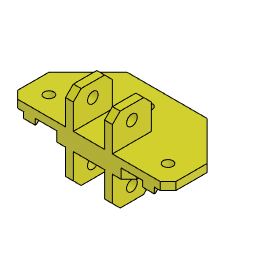
Bed Lift Idler Buddy_2x (Autodesk Fusion 360 design; units mm, degrees)
Autodesk Fusion 360 part; units mm, degrees
note: some values were not read from the file. Set by a fixed rule: the direction of a hole.
sketch "Sketch1" plane through (207.95, 134, 0) normal (0, 0, 1) x (1, 0, 0)
  line L0 (-207.95, -120) -> (-126.95, -120)
  line L1 (-126.95, -120) -> (-126.95, -134)
  line L2 (-126.95, -134) -> (-207.95, -134)
  line L3 (-207.95, -134) -> (-207.95, -120)
  line L4 (-167.45, -134) -> (-167.45, -146) construction
  line L5 (-167.45, -140) -> (-164.45, -140) construction
  line L6 (-167.45, -140) -> (-55.6884, -140)
  line L7 (-55.6884, -137.5) -> (-55.6884, -142.5)
  line L8 (-146.95, -120) -> (-146.95, -134)
  line L9 (-187.95, -120) -> (-187.95, -134)
  point P0 (-167.45, -134)
  point P1 (-207.95, -134)
  constraint horizontal L0
  constraint vertical L1
  constraint horizontal L2
  constraint vertical L3
  constraint midpoint L2 P0
  constraint vertical L4
  constraint coincident P0 L4.start
  constraint horizontal L5
  constraint midpoint L4 L5.start
  constraint perpendicular L4 L6
  constraint vertical L7
  constraint midpoint L6.end L7
  constraint coincident L0 L8.start
  constraint coincident L2 L8.end
  constraint perpendicular L2 L8
  constraint coincident L0 L9.start
  constraint coincident L2 L9.end
  constraint perpendicular L2 L9
  constraint coincident P1 L2.end
  measures "d6013" distance of L0.start L0.end
  measures "d6014" distance of L0.start L2.end
  measures "d6017" distance of P0 L4.end
  measures "d6018" distance of L5.start L5.end
  measures "d6019" distance of L7.start L7.end
  measures "d6020" distance of P1 L9.end
  measures "d6021" distance of L1.end L8.end
extrude "Extrude1" add sketch "Sketch1" along normal blind 4
extrude "Extrude2" add sketch "Sketch1" against normal blind 5 contours L0 L2 L8 L9
sketch "Sketch4" plane through (0, 14, 0) normal (0, 1, 0) x (-1, 0, 0)
  line L0 (-61, -5) -> (-20, -5)
  line L1 (-20, -5) -> (-20, 0)
  line L2 (-20, 0) -> (0, 0)
  line L3 (0, 4) -> (-81, 4)
  line L4 (-81, 0) -> (-61, 0)
  line L5 (-61, 0) -> (-61, -5)
  line L6 (0, 0) -> (0, 4)
  line L7 (-81, 4) -> (-81, 0)
  line L8 (-40.5, 4) -> (-40.5, -5) construction
  line L9 (-28.5, -22) -> (-52.5, -22)
  line L10 (-52.5, -22) -> (-52.5, -5)
  line L11 (-52.5, -5) -> (-28.5, -5)
  line L12 (-28.5, -5) -> (-28.5, -22)
  line L13 (-36.25, 234.1382) -> (-44.75, 234.1382) construction
  line L14 (-44.75, 234.1382) -> (-44.75, 246.1382) construction
  line L15 (-44.75, 246.1382) -> (-36.25, 246.1382) construction
  line L16 (-36.25, 246.1382) -> (-36.25, 234.1382) construction
  line L17 (-32.5, -22) -> (-32.5, -5)
  line L18 (-48.5, -5) -> (-48.5, -22)
  line L19 (-61, -0.5) -> (-20, -0.5) construction
  line L20 (-28.5, 4) -> (-28.5, 21)
  line L21 (-28.5, 21) -> (-52.5, 21)
  line L22 (-32.5, 21) -> (-32.5, 4)
  line L23 (-48.5, 4) -> (-48.5, 21)
  line L24 (-52.5, 21) -> (-52.5, 4)
  point P0 (-40.5, -0.5)
  point P1 (-40.5, -0.5)
  dimension "d6225" = 20
  dimension "d6226" = 17
  dimension "d6227" = 8.5
  dimension "d6228" = 12
  dimension "d6229" = 4
  dimension "d6280" = 22
  dimension "d576" = 16
  constraint midpoint L0 L8.end
  constraint midpoint L3 L8.start
  constraint horizontal L9
  constraint vertical L10
  constraint horizontal L11
  constraint vertical L12
  constraint symmetric L8 L9.start L9.end
  constraint horizontal L13
  constraint vertical L14
  constraint horizontal L15
  constraint vertical L16
  constraint symmetric L8 L13.start L13.end
  constraint coincident L9 L17.start
  constraint coincident L11 L17.end
  constraint perpendicular L11 L17
  constraint coincident L11 L18.start
  constraint coincident L9 L18.end
  constraint perpendicular L9 L18
  constraint symmetric L8 L17.start L18.end
  constraint coincident L0 L10.end
  constraint coincident L5 L19.start
  constraint coincident L1 L19.end
  constraint perpendicular L1 L19
  constraint midpoint L19 P1
  constraint midpoint L8 P1
  constraint coincident P1 P0
  constraint symmetric L9.start L19 L20.end
  constraint symmetric L9.end L19 L21.end
  constraint symmetric L10.end L19 L24.end
  constraint symmetric L11.end L19 L20.start
  constraint symmetric L17.start L19 L22.start
  constraint symmetric L17.end L19 L22.end
  constraint symmetric L18.start L19 L23.start
  constraint symmetric L18.end L19 L23.end
  measures "d6226" distance of L9.start L11.end
  measures "d6227" distance of L13.start L13.end
  measures "d6228" distance of L13.start L15.end
  measures "d6229" distance of L10.end L18.start
  measures "d6280" vertical distance of L4.end L9.end
  measures "d576" distance of L17.start L18.end
extrude "Extrude5" add sketch "Sketch4" along normal blind 3 and the other way blind 14 contours L0 L9 L10 L11 L18 | L0 L9 L11 L12 L17 | L3 L21 L23 L24 | L3 L20 L21 L22
hole "Hole5" at (28.5, 10, -15) direction (1, 0, 0) diameter 5.5 depth 55 tip angle 118
hole "Hole6" at (28.5, 10, 14) direction (1, 0, 0) diameter 5.5 depth 25 tip angle 118
sketch "Sketch5" plane through (28.5, 0, 0) normal (-1, 0, 0) x (0, -1, 0)
  circle A0 centre (-10, -15) radius 2.75
  line L0 (0, -5) -> (-14, -5)
  line L1 (-14, -5) -> (-17, -5)
  line L2 (-17, -5) -> (-17, -22)
  line L3 (-17, -22) -> (0, -22)
  line L4 (0, -22) -> (0, -5)
  circle A1 centre (-10, -15) radius 2.75
  circle A2 centre (-10, -15) radius 9 construction
  circle A3 centre (-10, -15) radius 6
  line L5 (-16, -15) -> (-16, 273.6321)
  line L6 (-16, 273.6321) -> (-14, 273.6321)
  line L7 (-14, 0) -> (-14, -5)
  line L8 (-10, -15) -> (-10, -22) construction
  dimension "d6290" = 18
  dimension "d6291" = 12
  dimension "d6292" = 2
  constraint concentric A0 A2
  constraint concentric A1 A3
  constraint coincident A3 L5.start
  constraint tangent A3 L5
  constraint perpendicular L1 L5
  constraint perpendicular L5 L6
  constraint coincident L6.end L7
  constraint coincident A0.centre A1.centre
  constraint coincident L3 L8.end
  constraint perpendicular L3 L8
  measures "d6290" diameter of A2
  measures "d6291" diameter of A3
  measures "d6292" distance of L5.end L6.end
sketch "Sketch6" plane through (0, 14, 0) normal (0, 1, 0) x (-1, 0, 0)
  line L0 (-20, 0) -> (0, 0)
  line L1 (0, 0) -> (0, 4)
  line L2 (0, 4) -> (-28.5, 4)
  line L3 (-28.5, 4) -> (-32.5, 4)
  line L4 (-52.5, 4) -> (-81, 4)
  line L5 (-81, 4) -> (-81, 0)
  line L6 (-81, 0) -> (-61, 0)
  line L7 (-61, 0) -> (-61, -5)
  line L8 (-61, -5) -> (-52.5, -5)
  line L9 (-52.5, -5) -> (-48.5, -5)
  line L10 (-48.5, -5) -> (-32.5, -5)
  line L11 (-32.5, -5) -> (-28.5, -5)
  line L12 (-28.5, -5) -> (-20, -5)
  line L13 (-20, -5) -> (-20, 0)
  line L14 (-61, 0) -> (-61, 4)
  line L15 (-20, 0) -> (-20, 4)
  line L16 (-32.5, 4) -> (-48.5, 4)
  line L17 (-48.5, 4) -> (-52.5, 4)
  constraint coincident L6.end L7.start
  constraint perpendicular L4 L14
  constraint coincident L0.start L13.end
  constraint perpendicular L2 L15
  constraint coincident L4 L14.end
  constraint coincident L2 L15.end
extrude "Extrude6" add sketch "Sketch6" along normal blind 6 contours L0 L1 L2 L15 | L4 L5 L6 L14
hole "Hole7" at (10, 10, 4) direction (0, 0, -1) diameter 5 depth 12 tip angle 180
hole "Hole8" at (71, 10, 4) direction (0, 0, -1) diameter 5 depth 10 tip angle 180
sketch "Sketch8" plane through (0, 20, 0) normal (0, 1, 0) x (-1, 0, 0)
  line L0 (0, 0) -> (0, 4)
  line L1 (0, 4) -> (-20, 4)
  line L2 (-20, 0) -> (0, 0)
  line L3 (-48.5, -5) -> (-48.5, -22)
  line L4 (-48.5, -22) -> (-52.5, -22)
  line L5 (-52.5, -22) -> (-52.5, -5)
  line L6 (-48.5, -5) -> (-32.5, -5)
  line L7 (-32.5, -22) -> (-32.5, -5)
  line L8 (-28.5, -5) -> (-28.5, -22)
  line L9 (-28.5, -22) -> (-32.5, -22)
  line L10 (-28.5, -5) -> (-20, -5)
  line L11 (-20, 0) -> (-20, -5)
  line L12 (-61, 0) -> (-61, -5)
  line L13 (-61, -5) -> (-52.5, -5)
  line L14 (-20, 0) -> (0, 0)
  line L15 (-81, 0) -> (-61, 0)
  line L16 (0, 0) -> (0, 4)
  line L17 (-81, 0) -> (-81, 4)
  line L18 (-10, 0) -> (-10, 4)
  line L19 (-71, 0) -> (-71, 5)
  line L20 (-74, 5) -> (-74, 10)
  line L21 (-74, 10) -> (-68, 10)
  line L22 (-68, 10) -> (-68, 5)
  line L23 (-13.0512, 4) -> (-13.0695, 9)
  line L24 (-7.0712, 9.1427) -> (-6.9488, 4)
  line L25 (-13.0695, 9) -> (-7.0712, 9.1427)
  line L26 (-20, -5) -> (-20, 4)
  line L27 (-24.25, -5) -> (-24.8161, 5.0059)
  line L28 (-61, -5) -> (-61, 5)
  line L29 (-56.75, -5) -> (-56.2231, 5.0071)
  line L30 (-20, 4) -> (-20, 0)
  line L31 (-32.5, 4) -> (-32.5, 21)
  line L32 (-32.5, 21) -> (-28.5, 21)
  line L33 (-28.5, 21) -> (-28.5, 4)
  line L34 (0, 4) -> (-28.5, 4)
  line L35 (-52.5, 4) -> (-52.5, 21)
  line L36 (-52.5, 21) -> (-48.5, 21)
  line L37 (-48.5, 21) -> (-48.5, 4)
  line L38 (-32.5, 4) -> (-48.5, 4)
  line L39 (-52.5, 4) -> (-81, 4)
  dimension "d6767" = 5
  dimension "d6768" = 5
  dimension "d6769" = 6
  dimension "d6770" = 6
  constraint midpoint L14 L18.start
  constraint midpoint L1 L18.end
  constraint midpoint L15 L19.start
  constraint perpendicular L20 L21
  constraint symmetric L19 L20.start L22.end
  constraint coincident L1 L24.end
  constraint symmetric L18 L23.start L24.end
  constraint perpendicular L24 L25
  constraint coincident L10.end L11.end
  constraint coincident L1.end L26.end
  constraint midpoint L10 L27.start
  constraint coincident L12.end L13.start
  constraint midpoint L13 L29.start
  measures "d6767" distance of L20.start L20.end
  measures "d6768" distance of L23.start L23.end
  measures "d6769" distance of L20.end L21.end
  measures "d6770" distance of L23.end L24.start
extrude "Extrude8" add sketch "Sketch8" against normal blind 6 contours L10 L11 L26 L27 L30 L34 | L12 L13 L28 L29 L39
sketch "Sketch9" plane through (0, 0, 0) normal (0, 0, -1) x (1, 0, 0)
  circle A0 centre (71, -10) radius 2.5
  line L0 (61, 0) -> (61, -20)
  line L1 (61, -20) -> (81, -20)
  line L2 (81, -20) -> (81, 0)
  line L3 (81, 0) -> (61, 0)
  circle A1 centre (10, -10) radius 2.5
  line L4 (20, -20) -> (20, 0)
  line L5 (20, 0) -> (0, 0)
  line L6 (0, 0) -> (0, -20)
  line L7 (0, -20) -> (20, -20)
  line L8 (81, -20) -> (81, -40)
  line L9 (81, -40) -> (61, -40)
  line L10 (61, -40) -> (61, -20)
  line L11 (0, -20) -> (0, -40)
  line L12 (0, -40) -> (20, -40)
  line L13 (20, -40) -> (20, -20)
  line L14 (20, -40) -> (81, -40)
  line L15 (81, -40) -> (81, 0)
  line L16 (81, 0) -> (20, 0)
  line L17 (20, 0) -> (20, -40)
  dimension "d305" = 20
  constraint coincident L1.end L2.start
  constraint perpendicular L1 L8
  constraint perpendicular L2 L9
  constraint coincident L0.end L1.start
  constraint perpendicular L1 L10
  constraint coincident L6.end L7.start
  constraint perpendicular L7 L11
  constraint perpendicular L4 L12
  constraint coincident L4.start L7.end
  constraint perpendicular L12 L13
  constraint equal L10 L13
  constraint horizontal L14
  constraint vertical L15
  constraint horizontal L16
  constraint vertical L17
  constraint coincident L2.end L3.start
  measures "d305" distance of L12.end L4.start
extrude "Extrude9" add sketch "Sketch9" against normal blind 4 contours L0 L4 L10 L13 L14 L16 L17 | L1 L8 L9 L10 L14 L15 | L7 L11 L12 L13 L17
hole "Hole9" at (40.469, 30, 0) direction (0, 0, 1) diameter 5 depth 16 tip angle 118
extrude "Extrude10" add 1 faces at (43.1732, 14, -1.6667) along direction (0, 1, 0) blind 6
extrude "Extrude11" add 4 faces at (51.1667, 17, 9.6667) (29.8333, 17, 15.3333) (29.8333, 17, -16.3333) (51.1667, 17, -10.6667) along direction (0, 1, 0) blind 3
chamfer "Chamfer7" distance 4 angle 45 14 edges at (50.5, 0, 21) (30.5, 0, 21) (30.5, 0, -22) (50.5, 0, -22) (50.5, 20, 21) (30.5, 20, 21) (30.5, 20, -22) (50.5, 20, -22) (0, 0, 2) (81, 0, 2) (61, 20, -2.5) (20, 20, -2.5) (61, 0, -2.5) (20, 0, -2.5)
chamfer "Chamfer12" distance 20 angle 45 2 edges at (0, 40, 2) (81, 40, 2)
sketch "Sketch11" plane through (0, 0, 0) normal (0, -1, 0) x (1, 0, 0)
  line L0 (24, 0) -> (24, -5)
  line L1 (24, -5) -> (28.5, -5)
  line L2 (28.5, -5) -> (28.5, -18)
  line L3 (28.5, -18) -> (32.5, -18)
  line L4 (32.5, -18) -> (32.5, -5)
  line L5 (32.5, -5) -> (48.5, -5)
  line L6 (48.5, -5) -> (48.5, -18)
  line L7 (48.5, -18) -> (52.5, -18)
  line L8 (52.5, -18) -> (52.5, -5)
  line L9 (52.5, -5) -> (57, -5)
  line L10 (57, -5) -> (57, 0)
  line L11 (57, 0) -> (77, 0)
  line L12 (77, 0) -> (77, 4)
  line L13 (77, 4) -> (52.5, 4)
  line L14 (52.5, 4) -> (52.5, 17)
  line L15 (52.5, 17) -> (48.5, 17)
  line L16 (48.5, 17) -> (48.5, 4)
  line L17 (48.5, 4) -> (32.5, 4)
  line L18 (32.5, 4) -> (32.5, 17)
  line L19 (32.5, 17) -> (28.5, 17)
  line L20 (28.5, 17) -> (28.5, 4)
  line L21 (28.5, 4) -> (4, 4)
  line L22 (4, 4) -> (4, 0)
  line L23 (4, 0) -> (24, 0)
  line L24 (12.5, 0) -> (7.5, 0)
  line L25 (7.5, 4) -> (12.5, 4)
  line L26 (73.5, 0) -> (68.5, 0)
  line L27 (68.5, 4) -> (73.5, 4)
  line L28 (10, 0) -> (10, -3) construction
  line L29 (10, -3) -> (71, -3) construction
  line L30 (71, -3) -> (71, 0) construction
  line L31 (7, 0) -> (13, 0)
  line L32 (13, 0) -> (13, -3)
  line L33 (13, -3) -> (7, -3)
  line L34 (7, -3) -> (7, 0)
  line L35 (74, 0) -> (68, 0)
  line L36 (68, 0) -> (68, -3)
  line L37 (68, -3) -> (74, -3)
  line L38 (74, -3) -> (74, 0)
  dimension "d916" = 3
  dimension "d917" = 6
  dimension "d918" = 6
  constraint midpoint L24 L28.start
  constraint perpendicular L24 L28
  constraint perpendicular L4 L29
  constraint midpoint L26 L30.end
  constraint perpendicular L26 L30
  constraint horizontal L31
  constraint vertical L32
  constraint horizontal L33
  constraint vertical L34
  constraint coincident L24 L31.start
  constraint horizontal L35
  constraint vertical L36
  constraint horizontal L37
  constraint vertical L38
  constraint coincident L26 L35.start
  constraint midpoint L29.end L37
  constraint midpoint L28.end L33
  measures "d916" distance of L29.end L30.end
  measures "d917" distance of L32.end L33.end
  measures "d918" distance of L36.end L37.end
extrude "Extrude12" add sketch "Sketch11" against normal blind 20 contours L23 L24 L31 L32 L33 L34 | L11 L26 L35 L36 L37 L38
sketch "Sketch12" plane through (0, 0, -3) normal (0, 0, -1) x (1, 0, 0)
  line L0 (13, 0) -> (7, 0)
  line L1 (7, 0) -> (7, -20)
  line L2 (7, -20) -> (13, -20)
  line L3 (13, -20) -> (13, 0)
  line L4 (74, 0) -> (68, 0)
  line L5 (68, 0) -> (68, -20)
  line L6 (68, -20) -> (74, -20)
  line L7 (74, -20) -> (74, 0)
  circle A0 centre (71, -10) radius 2.5 construction
  circle A1 centre (10, -10) radius 2.5 construction
  line L8 (74, -17.5) -> (68, -17.5)
  line L9 (68, -17.5) -> (68, -2.5)
  line L10 (68, -2.5) -> (74, -2.5)
  line L11 (74, -2.5) -> (74, -17.5)
  line L12 (74, -17.5) -> (68, -2.5) construction
  line L13 (68, -17.5) -> (74, -2.5) construction
  line L14 (13, -17.5) -> (7, -17.5)
  line L15 (7, -17.5) -> (7, -2.5)
  line L16 (7, -2.5) -> (13, -2.5)
  line L17 (13, -2.5) -> (13, -17.5)
  line L18 (13, -17.5) -> (7, -2.5) construction
  line L19 (7, -17.5) -> (13, -2.5) construction
  point P0 (71, -10)
  point P1 (10, -10)
  dimension "d924" = 15
  dimension "d925" = 15
  constraint horizontal L8
  constraint perpendicular L8 L9
  constraint parallel L8 L10
  constraint parallel L9 L11
  constraint coincident L7 L8.start
  constraint coincident L12 P0
  constraint coincident L13 P0
  constraint coincident P0 A0.centre
  constraint horizontal L14
  constraint perpendicular L14 L15
  constraint parallel L14 L16
  constraint parallel L15 L17
  constraint coincident L3 L14.start
  constraint coincident L18 P1
  constraint coincident L19 P1
  constraint coincident P1 A1.centre
  measures "d924" distance of L14.start L16.end
  measures "d925" distance of L8.start L10.end
extrude "Extrude14" cut sketch "Sketch12" against normal up to surface (3 mm away) contours L1 L3 L14 L15 L16 L17 | L5 L7 L8 L9 L10 L11
chamfer "Chamfer13" distance 2 angle 45 4 edges at (10, 17.5, -3) (71, 17.5, -3) (10, 2.5, -3) (71, 2.5, -3)
chamfer "Chamfer14" distance 1 angle 45 2 edges at (10, 17.5, 0) (71, 17.5, 0)
equation "d6768 = d6767"
equation "d6770 = d6769"
equation "d576 = 12.00 mm + 4 mm"
equation "d918 = d917"
equation "d925 = d924"
named bodies: "11mm Bed Lift Buddy_2x_SN_BY"
